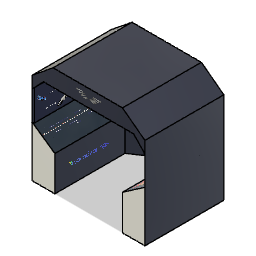
f1-pit-display-radtek (Autodesk Fusion 360 design; units mm, degrees)
Autodesk Fusion 360 part; units mm, degrees
sketch "Sketch1" plane through (0, 0, 0) normal (0, 1, 0) x (1, 0, 0)
  line L0 (-50, 50) -> (50, 50)
  line L1 (50, 50) -> (50, -50)
  line L2 (50, -50) -> (-50, -50)
  line L3 (-50, -50) -> (-50, 50)
  constraint horizontal L0
  constraint perpendicular L0 L1
  constraint perpendicular L1 L2
  constraint perpendicular L2 L3
extrude "Extrude1" add sketch "Sketch1" along normal blind 31 makes body 1
sketch "Sketch2" plane through (0, 31, 0) normal (0, 1, 0) x (-1, 0, 0)
  line L0 (50, 50) -> (-50, 50)
  line L1 (-50, 50) -> (-50, -50)
  line L2 (-50, -50) -> (50, -50)
  line L3 (50, -50) -> (50, 50)
  line L4 (-105, 50) -> (-75, 20)
  line L5 (-75, 20) -> (-75, -30)
  line L6 (-75, -30) -> (-105, -50)
  line L7 (-175, 20) -> (-175, -30)
  line L8 (-175, -30) -> (-145, -50)
  line L9 (-145, -50) -> (-105, -50)
  line L10 (-175, 20) -> (-145, 50)
  line L11 (-105, 50) -> (-145, 50)
  constraint perpendicular L2 L5
  constraint parallel L5 L7
  constraint perpendicular L7 L9
  constraint horizontal L11
extrude "Extrude2" add sketch "Sketch2" along normal blind 50 thin wall 1 inside separate body contours L4 L5 L6 L7 L8 L9 L10 L11 makes body 2
sketch "Sketch3" plane through (0, 81, 0) normal (0, 1, 0) x (-1, 0, 0)
sketch "Sketch4" plane through (0, 0, 50) normal (0, 0, 1) x (1, 0, 0)
  line L0 (105, 31) -> (145, 31)
  line L1 (145, 31) -> (145, 81)
  line L2 (145, 81) -> (105, 81)
  line L3 (105, 81) -> (105, 31)
  line L4 (105, 81) -> (105, 31)
  line L5 (145, 31) -> (105, 31)
  line L6 (145, 31) -> (145, 81)
  line L7 (145, 81) -> (105, 81)
  constraint coincident L2.end L3.start
  constraint coincident L0.start L3.end
  constraint coincident L0.end L1.start
  constraint coincident L1.end L2.start
extrude "Extrude3" cut sketch "Sketch4" against normal blind 30 bodies 2
extrude "Extrude4" cut 1 faces at (165, 64.3333, 30) along direction (-0.707107, 0, -0.707107) blind 20 on bodies 2 bodies 2
extrude "Extrude5" cut 1 faces at (95, 47.6667, 40) along direction (0.707107, 0, -0.707107) blind 5 on bodies 2 bodies 2
move_body "Move1" bodies 2 to x (1, 0, 0) y (0, 1, 0) z (0, 0, 1) at (-125, 0, 0)
sketch "Sketch5" plane through (0, 31, 0) normal (0, 1, 0) x (-1, 0, 0)
  line L0 (50, 50) -> (-50, 50)
  line L1 (-50, 50) -> (-50, -50)
  line L2 (-50, -50) -> (50, -50)
  line L3 (50, -50) -> (50, 50)
sketch "Sketch6" plane through (0, 31, 0) normal (0, 1, 0) x (-1, 0, 0)
  line L0 (50, 20) -> (-50, 20)
  line L1 (50, 20) -> (50, 50)
  line L2 (50, 50) -> (-50, 50)
  line L3 (-50, 50) -> (-50, 20)
  constraint horizontal L0
  constraint perpendicular L0 L1
  constraint perpendicular L1 L2
  constraint perpendicular L0 L3
extrude "Extrude6" cut sketch "Sketch6" against normal blind 100 bodies 1
sketch "Sketch7" plane through (0, 31, 0) normal (0, 1, 0) x (-1, 0, 0)
  line L0 (20, -50) -> (50, -50)
  line L1 (50, -50) -> (50, -30)
  line L2 (50, -30) -> (20, -50)
  constraint horizontal L0
  constraint perpendicular L0 L1
extrude "Extrude7" add sketch "Sketch7" along normal blind 50 bodies 1 2
sketch "Sketch8" plane through (0, 31, 0) normal (0, 1, 0) x (-1, 0, 0)
  line L0 (-50, -30) -> (-50, -50)
  line L1 (-50, -50) -> (-20, -50)
  line L2 (-20, -50) -> (-50, -30)
  constraint vertical L0
  constraint perpendicular L0 L1
extrude "Extrude8" add sketch "Sketch8" along normal blind 50 bodies 1
sketch "Sketch9" plane through (0, 0, 20) normal (0, 0, 1) x (1, 0, 0)
  line L0 (-50, 0) -> (50, 0)
  line L1 (50, 0) -> (50, 31)
  line L2 (50, 31) -> (-50, 31)
  line L3 (-50, 31) -> (-50, 0)
  line L4 (-50, 31) -> (-50, 45)
  line L5 (-50, 45) -> (-29.8494, 31)
  line L6 (-29.8494, 31) -> (-50, 31)
  line L7 (-50, 31) -> (-29.8494, 31)
  constraint coincident L2.end L3.start
  constraint perpendicular L2 L4
  constraint coincident L2 L5.end
extrude "Extrude9" add sketch "Sketch9" against normal blind 65 contours L2 L4 L5 L6 L7 bodies 1
sketch "Sketch10" plane through (0, 0, 20) normal (0, 0, 1) x (1, 0, 0)
  line L0 (-50, 0) -> (50, 0)
  line L1 (50, 0) -> (50, 31)
  line L2 (50, 31) -> (-29.8494, 31)
  line L3 (-29.8494, 31) -> (-50, 45)
  line L4 (-50, 45) -> (-50, 0)
  line L5 (50, 31) -> (50, 45)
  line L6 (50, 45) -> (29.8584, 31)
  line L7 (50, 31) -> (29.8584, 31)
  constraint coincident L1.end L2.start
  constraint perpendicular L2 L5
  constraint coincident L2 L6.end
extrude "Extrude10" add sketch "Sketch10" against normal blind 70 contours L2 L5 L6 L7 bodies 1
sketch "Sketch11" plane through (0, 81, 0) normal (0, 1, 0) x (-1, 0, 0)
  line L0 (50, 20) -> (49, 19)
  line L1 (49, 19) -> (49, -29.4648)
  line L2 (49, -29.4648) -> (19.6972, -49)
  line L3 (19.6972, -49) -> (-19.6972, -49)
  line L4 (-19.6972, -49) -> (-49, -29.4648)
  line L5 (-49, -29.4648) -> (-49, 19)
  line L6 (-49, 19) -> (-50, 20)
  line L7 (-50, 20) -> (-50, -50)
  line L8 (-50, -50) -> (50, -50)
  line L9 (50, -50) -> (50, 20)
  line L10 (50, -50) -> (-50, -50)
  line L11 (-50, -50) -> (-50, 20)
  line L12 (50, -50) -> (50, 20)
  line L13 (50, 20) -> (-50, 20)
  constraint coincident L8.end L9.start
  constraint coincident L7.end L8.start
  constraint coincident L6.end L7.start
  constraint coincident L0.start L9.end
extrude "Extrude11" add sketch "Sketch11" along normal blind 15 separate body contours L0 L1 L2 L3 L4 L5 L6 L13 makes body 3
sketch "Sketch12" plane through (0, 0, 20) normal (0, 0, 1) x (1, 0, 0)
  line L0 (-50, 81) -> (50, 81)
  line L1 (50, 81) -> (50, 96)
  line L2 (50, 96) -> (-50, 96)
  line L3 (-50, 96) -> (-50, 81)
  line L4 (-50, 81) -> (-31.4553, 96)
  line L5 (-50, 81) -> (-50, 96)
  line L6 (-50, 96) -> (-31.4553, 96)
  constraint coincident L0.start L3.end
  constraint coincident L2 L4.end
  constraint coincident L2.end L3.start
sketch "Sketch13" plane through (0, 81, 0) normal (0, 1, 0) x (-1, 0, 0)
  line L0 (50, 20) -> (49, 19)
  line L1 (49, 19) -> (49, -29.4648)
  line L2 (49, -29.4648) -> (19.6972, -49)
  line L3 (19.6972, -49) -> (-19.6972, -49)
  line L4 (-19.6972, -49) -> (-49, -29.4648)
  line L5 (-49, -29.4648) -> (-49, 19)
  line L6 (-49, 19) -> (-50, 20)
  line L7 (-50, 20) -> (-50, -50)
  line L8 (-50, -50) -> (50, -50)
  line L9 (50, -50) -> (50, 20)
  line L10 (49, -29.4648) -> (50, -29.4648)
  line L11 (50, -29.4648) -> (50, 20)
  line L12 (50, 20) -> (49, 19)
  line L13 (49, 19) -> (49, -29.4648)
  line L14 (49, 19) -> (49, -29.4648)
  constraint coincident L1.end L2.start
  constraint coincident L9 L10.end
  constraint perpendicular L9 L10
  constraint coincident L0.start L9.end
  constraint coincident L0.end L1.start
extrude "Extrude12" add sketch "Sketch13" along normal blind 20 contours L0 L1 L9 L10 L11 L12 L13 L14 bodies 1 3
extrude "Extrude13" add 1 faces at (-39.5657, 81, -42.8216) along direction (0, 1, 0) blind 15 on bodies 1 bodies 1
extrude "Extrude14" cut sketch "Sketch12" against normal blind 115 contours L2 L3 L4 L5 L6 bodies 1 makes body 4 at (-50, 97.6667, 3.5117)
sketch "Sketch14" plane through (0, 0, 20) normal (0, 0, 1) x (1, 0, 0)
  line L0 (-31.4553, 96) -> (-50, 81)
  line L1 (-50, 81) -> (50, 81)
  line L2 (50, 81) -> (50, 96)
  line L3 (50, 96) -> (-31.4553, 96)
  line L4 (50, 81) -> (30.0924, 96)
  line L5 (30.0924, 96) -> (50, 96)
  line L6 (50, 96) -> (50, 81)
  constraint coincident L1.end L2.start
  constraint coincident L3 L4.end
  constraint coincident L2.end L3.start
  constraint perpendicular L2 L5
extrude "Extrude15" cut sketch "Sketch14" against normal blind 110 contours L2 L3 L4 L5 L6 bodies 1
sketch "Sketch15" plane through (-50, 0, 0) normal (-1, 0, 0) x (0, 0, 1)
  line L0 (20, 81) -> (-50, 81)
  line L1 (-50, 81) -> (-50, 0)
  line L2 (-50, 0) -> (20, 0)
  line L3 (20, 0) -> (20, 45)
  line L4 (20, 45) -> (20, 81)
sketch "Sketch16" plane through (0, 0, 20) normal (0, 0, 1) x (1, 0, 0)
  line L0 (50, 81) -> (30.0924, 96)
  line L1 (30.0924, 96) -> (-31.4553, 96)
  line L2 (-31.4553, 96) -> (-50, 81)
  line L3 (-50, 81) -> (50, 81)
  line L4 (-50, 81) -> (-50, 70.4953)
  line L5 (-50, 70.4953) -> (-40, 81)
  line L6 (-50, 81) -> (-40, 81)
  line L7 (50, 81) -> (50, 70.4953)
  line L8 (50, 70.4953) -> (40, 81)
  line L9 (40, 81) -> (50, 81)
  constraint coincident L2.end L3.start
  constraint perpendicular L3 L4
  constraint coincident L3 L5.end
  constraint coincident L0.start L3.end
  constraint perpendicular L3 L7
  constraint coincident L3 L8.end
extrude "Extrude16" add sketch "Sketch16" against normal blind 70 contours L3 L7 L8 L9 | L3 L4 L5 L6 bodies 1
sketch "Sketch17" plane through (-50, 0, 0) normal (-1, 0, 0) x (0, 0, 1)
  line L0 (-50, 81) -> (20, 81)
  line L1 (20, 81) -> (20, 0)
  line L2 (20, 0) -> (-50, 0)
  line L3 (-50, 0) -> (-50, 81)
  constraint horizontal L0
  constraint vertical L1
  constraint horizontal L2
  constraint vertical L3
sketch "Sketch18" plane through (0, 31, 0) normal (0, 1, 0) x (-1, 0, 0)
  line L0 (-29.8584, 20) -> (-29.8584, -42.2259)
  line L1 (-29.8584, -42.2259) -> (-19.6972, -49)
  line L2 (-19.6972, -49) -> (19.6972, -49)
  line L3 (19.6972, -49) -> (29.8494, -42.2319)
  line L4 (29.8494, -42.2319) -> (29.8494, 20)
  line L5 (29.8494, 20) -> (-29.8584, 20)
  line L6 (29.8494, 20) -> (29.8494, -42.2319)
  line L7 (29.8494, -42.2319) -> (19.6972, -49)
  line L8 (19.6972, -49) -> (-19.6972, -49)
  line L9 (-19.6972, -49) -> (-29.8584, -42.2259)
  line L10 (-29.8584, -42.2259) -> (-29.8584, 20)
  line L11 (-29.8584, 20) -> (29.8494, 20)
  constraint coincident L4.end L5.start
  constraint coincident L3.end L4.start
  constraint coincident L2.end L3.start
  constraint coincident L1.end L2.start
  constraint coincident L0.end L1.start
  constraint coincident L0.start L5.end
extrude "Extrude17" cut sketch "Sketch18" against normal blind 60 bodies 1
hidden bodies 4
